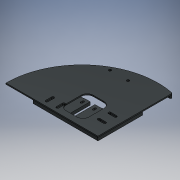
# Autodesk Inventor part: D0001
Saved by Autodesk Inventor 2017 (Build 210142000, 142)
## iProperties
Part Number: D0001
Material: SS41
Document SubType Name: Modeling
Designer: G
Density: 7.85 g/cm^3
Appearance: 鐵灰色
Author: G
Autodesk Inventor part; units mm, degrees
ref_plane "YZ Plane" through (0, 0, 0) normal (1, 0, 0) x (0, 1, 0)
ref_plane "XZ Plane" through (0, 0, 0) normal (0, 1, 0) x (-1, 0, 0)
ref_plane "XY Plane" through (0, 0, 0) normal (0, 0, 1) x (1, 0, 0)
sketch "草圖1" plane through (0, 0, 0) normal (0, 0, 1) x (1, 0, 0)
  arc A0 (0, 45) -> (-45, 0) centre (0, 0) ccw
  arc A1 (0, 65) -> (-65, 0) centre (0, 0) ccw
  line L0 (0, 65) -> (0, 0)
  line L1 (0, 0) -> (-65, 0)
  arc A2 (18, 45) -> (60.0968, 74.0984) centre (18, 90) ccw
  line L2 (0, 0) -> (63, 0)
  line L3 (63, 73.5683) -> (63, 0)
  arc A3 (63, 73.5683) -> (60.0968, 74.0984) centre (61.5, 73.5683) ccw
  line L4 (13, 45) -> (13, 10)
  line L5 (13, 10) -> (5, 10)
  line L6 (5, 10) -> (5, 45)
  line L7 (0, 45) -> (5, 45)
  line L8 (13, 45) -> (18, 45)
  line L9 (39.3, 43) -> (49.3, 43) construction
  line L10 (39.3, 40.9) -> (49.3, 40.9)
  line L11 (49.3, 45.1) -> (39.3, 45.1)
  arc A4 (39.3, 45.1) -> (39.3, 40.9) centre (39.3, 43) ccw
  arc A5 (49.3, 40.9) -> (49.3, 45.1) centre (49.3, 43) ccw
  line L12 (39.3, 25) -> (49.3, 25) construction
  line L13 (39.3, 22.9) -> (49.3, 22.9)
  line L14 (49.3, 27.1) -> (39.3, 27.1)
  arc A6 (39.3, 27.1) -> (39.3, 22.9) centre (39.3, 25) ccw
  arc A7 (49.3, 22.9) -> (49.3, 27.1) centre (49.3, 25) ccw
  line L15 (-30, 18) -> (-30, 8) construction
  line L16 (-32.1, 18) -> (-32.1, 8)
  line L17 (-27.9, 8) -> (-27.9, 18)
  arc A8 (-27.9, 18) -> (-32.1, 18) centre (-30, 18) ccw
  arc A9 (-32.1, 8) -> (-27.9, 8) centre (-30, 8) ccw
  line L18 (-12, 18) -> (-12, 8) construction
  line L19 (-14.1, 18) -> (-14.1, 8)
  line L20 (-9.9, 8) -> (-9.9, 18)
  arc A10 (-9.9, 18) -> (-14.1, 18) centre (-12, 18) ccw
  arc A11 (-14.1, 8) -> (-9.9, 8) centre (-12, 8) ccw
  point P0 (44.3, 43)
  point P1 (44.3, 25)
  point P2 (-30, 13)
  point P3 (-12, 13)
  dimension "d0" = 20
  dimension "d7" = 1.5
  dimension "d11" = 10
  dimension "d12" = 8
  dimension "d15" = 5
  dimension "d16" = 5
  dimension "d17" = 35
  dimension "d24" = 45
  dimension "d67" = 10
  dimension "d68" = 2.1
  dimension "d69" = 18
  dimension "d70" = 25
  dimension "d71" = 18.7
  dimension "d72" = 18
  dimension "d73" = 75
  dimension "d74" = 8
  constraints: 50 end point, 24 point on circle, 21 tangent, 12 centre point, 6 parallel, 5 horizontal, 4 midpoint, 4 vertical, 3 equal length, 3 equal radius, 2 coincident, 2 point on line, 1 horizontal alignment, 1 perpendicular, 1 vertical alignment
  measures "d0" radial gap between concentric circles of A0 A1
  measures "d7" radius of A3
  measures "d11" distance between parallel lines of L2 L5
  measures "d12" distance between parallel lines of L6 L4
  measures "d15" distance from line of L6 L7.start
  measures "d16" distance of L4.start L8.end
  measures "d17" distance of L4.start L4.end
  measures "d24" radius of A2
  measures "d67" distance of L11.start L11.end
  measures "d68" radius of A4
  measures "d69" distance between parallel lines of L12 L9
  measures "d70" distance between parallel lines of L2 L12
  measures "d71" distance from line of L3 point (44.3, 25)
  measures "d72" distance between parallel lines of L18 L15
  measures "d73" distance between parallel lines of L3 L18
  measures "d74" distance from line of L1 L15.end
extrude "擠出1" add sketch "草圖1" along normal mid plane 5 contours L0 L1 A0 | L7 L6 L5 L4 L8 A2 A3 L3 L2 L0
sketch "草圖3" plane through (0, 0, 2.5) normal (0, 0, 1) x (1, 0, 0)
  line L0 (-1.6, 39.7) -> (-0.5, 39.7) construction
  arc A0 (-0.5, 36.5) -> (-0.5, 39.7) centre (-0.5, 38.1) ccw construction
  line L1 (18.5, 39.7) -> (19.6, 39.7) construction
  line L2 (-1.05, 39.6) -> (-1.05, 36.6) construction
  line L3 (-2.65, 39.6) -> (-2.65, 36.6)
  line L4 (0.55, 36.6) -> (0.55, 39.6)
  arc A1 (0.55, 39.6) -> (-2.65, 39.6) centre (-1.05, 39.6) ccw
  arc A2 (-2.65, 36.6) -> (0.55, 36.6) centre (-1.05, 36.6) ccw
  line L5 (19.05, 39.6) -> (19.05, 36.6) construction
  line L6 (17.45, 39.6) -> (17.45, 36.6)
  line L7 (20.65, 36.6) -> (20.65, 39.6)
  arc A3 (20.65, 39.6) -> (17.45, 39.6) centre (19.05, 39.6) ccw
  arc A4 (17.45, 36.6) -> (20.65, 36.6) centre (19.05, 36.6) ccw
  point P0 (0, 0)
  point P1 (-1.05, 38.1)
  point P2 (19.05, 38.1)
  point P3 (-1.05, 39.7)
  point P4 (19.05, 39.7)
  dimension "d18" = 3.2
  dimension "d19" = 3.2
  dimension "d20" = 3
  dimension "d21" = 3
  constraints: 16 end point, 8 point on circle, 8 tangent, 4 centre point, 4 midpoint, 3 parallel, 2 horizontal alignment, 2 vertical alignment, 1 perpendicular
  measures "d18" distance between parallel lines of L4 L3
  measures "d19" distance between parallel lines of L7 L6
  measures "d20" distance of L3.start L3.end
  measures "d21" distance of L6.start L6.end
extrude "擠出3" cut sketch "草圖3" along normal through all both and the other way through all
sketch "草圖4" plane through (0, 0, 0) normal (0, 0, 1) x (1, 0, 0)
  circle A0 centre (104.6897, 76.6524) radius 22.5
  arc A1 (18, 45) -> (60.0968, 74.0984) centre (18, 90) ccw construction
  arc A2 (0, 45) -> (-45, 0) centre (0, 0) ccw construction
  line L0 (63, 73.5683) -> (63, 0) construction
  line L1 (63, 73.5683) -> (63, 177.2446) construction
  arc A3 (63, 120.0271) -> (38.7191, 113.6922) centre (61.7694, 75.0439) ccw construction
  line L2 (63, 0) -> (-45, 0) projected
  circle A4 centre (-22, 105) radius 2.1
  circle A5 centre (8, 105) radius 2.1
  line L3 (-22, 105) -> (8, 105) construction
  line L4 (-7, 105) -> (-7, 104.6648) construction
  arc A6 (63, 73.5683) -> (60.0968, 74.0984) centre (61.5, 73.5683) ccw construction
  arc A7 (61.4565, 121.0001) -> (22.4402, 102.0912) centre (60.0968, 74.0984) ccw
  arc A8 (-1.2272, 89.9916) -> (22.4402, 102.0912) centre (-1.6363, 119.9888) ccw
  arc A9 (0, 45) -> (-45, 0) centre (0, 0) ccw projected
  line L5 (-45, 0) -> (-90, 0) construction
  arc A10 (-1.2272, 89.9916) -> (-79.7772, 41.6604) centre (0, 0) ccw
  arc A11 (61.7997, 123.9692) -> (-82.5182, 42.8629) centre (36.5204, 0) ccw
  arc A12 (61.4565, 121.0001) -> (61.7997, 123.9692) centre (61.5, 122.4994) ccw
  arc A13 (-82.5182, 42.8629) -> (-79.7772, 41.6604) centre (-81.1069, 42.3548) ccw
  dimension "d25" = 45
  dimension "d28" = 45
  dimension "d35" = 30
  dimension "d36" = 4.2
  dimension "d56" = 45
  dimension "d58" = 30
  dimension "d61" = 55
  dimension "d62" = 105
  constraints: 18 point on circle, 10 centre point, 9 tangent, 8 end point, 4 equal radius, 2 coincident, 2 horizontal, 1 midpoint, 1 perpendicular, 1 point on line, 1 vertical, 1 other
  measures "d25" diameter of A0
  measures "d28" radius of A3
  measures "d35" distance of L3.end L3.start
  measures "d36" diameter of A4
  measures "d56" distance of L2.end L5.end
  measures "d58" radius of A8
  measures "d61" distance from line of L3.end L0
  measures "d62" distance between parallel lines of L2 L3
extrude "擠出4" add sketch "草圖4" against normal up to surface (5 mm away) from surface at 2.5 separate body contours A7 A8 A10 A13 A11 A12
sketch "草圖5" plane through (0, 0, 2.5) normal (0, 0, 1) x (1, 0, 0)
  arc A0 (18, 45) -> (60.0968, 74.0984) centre (18, 90) ccw construction
  line L0 (18, 45) -> (13, 45) construction
  line L1 (5, 45) -> (0, 45) construction
  arc A1 (0, 45) -> (-45, 0) centre (0, 0) ccw construction
  line L2 (5, 45) -> (13, 45) construction
  line L3 (-90, 0) -> (63, 0)
  line L4 (63, 122.4994) -> (63, 0)
  line L5 (0, 55) -> (18, 55)
  line L6 (28, 45) -> (28, 20)
  line L7 (18, 10) -> (0, 10)
  line L8 (-10, 20) -> (-10, 45)
  line L9 (13, 10) -> (5, 10) construction
  arc A2 (0, 55) -> (-10, 45) centre (0, 45) ccw
  arc A3 (28, 45) -> (18, 55) centre (18, 45) ccw
  arc A4 (18, 10) -> (28, 20) centre (18, 20) ccw
  arc A5 (-10, 20) -> (0, 10) centre (0, 20) ccw
  circle A6 centre (-22, 105) radius 2.1 projected
  circle A7 centre (8, 105) radius 2.1 projected
  arc A8 (61.7997, 123.9692) -> (-82.5182, 42.8629) centre (36.5204, 0) ccw projected
  arc A9 (-82.5182, 42.8629) -> (-90, 0) centre (36.5204, 0) ccw
  arc A10 (63, 122.4994) -> (61.7997, 123.9692) centre (61.5, 122.4994) ccw
  line L10 (49.3, 40.9) -> (39.3, 40.9) projected
  arc A11 (39.3, 45.1) -> (39.3, 40.9) centre (39.3, 43) ccw projected
  line L11 (39.3, 45.1) -> (49.3, 45.1) projected
  arc A12 (49.3, 40.9) -> (49.3, 45.1) centre (49.3, 43) ccw projected
  line L12 (39.3, 27.1) -> (49.3, 27.1) projected
  arc A13 (39.3, 27.1) -> (39.3, 22.9) centre (39.3, 25) ccw projected
  line L13 (49.3, 22.9) -> (39.3, 22.9) projected
  arc A14 (49.3, 22.9) -> (49.3, 27.1) centre (49.3, 25) ccw projected
  arc A15 (-27.9, 18) -> (-32.1, 18) centre (-30, 18) ccw projected
  line L14 (-32.1, 8) -> (-32.1, 18) projected
  arc A16 (-32.1, 8) -> (-27.9, 8) centre (-30, 8) ccw projected
  line L15 (-27.9, 18) -> (-27.9, 8) projected
  arc A17 (-9.9, 18) -> (-14.1, 18) centre (-12, 18) ccw projected
  line L16 (-14.1, 8) -> (-14.1, 18) projected
  line L17 (-9.9, 18) -> (-9.9, 8) projected
  arc A18 (-14.1, 8) -> (-9.9, 8) centre (-12, 8) ccw projected
  point P0 (-10, 55)
  point P1 (28, 55)
  point P2 (9, 10)
  point P3 (-21.8569, 69.1091)
  dimension "d41" = 38
  dimension "d42" = 10
  dimension "d45" = 10
  dimension "d47" = 45
  constraints: 15 point on circle, 14 end point, 11 tangent, 6 centre point, 5 point on line, 3 equal radius, 3 horizontal, 2 midpoint, 2 parallel, 2 perpendicular, 1 coincident
  measures "d41" distance of point (-10, 55) point (28, 55)
  measures "d42" radius of A2
  measures "d45" distance between parallel lines of L2 L5
  measures "d47" distance of A1.end L3.start
extrude "擠出5" add sketch "草圖5" along normal blind 2 separate body
